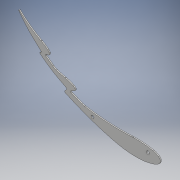
# Autodesk Inventor part: splitter
Saved by Autodesk Inventor 2018.3 (Build 223284000, 284)
## iProperties
Created: 2018-06-13
Part Number: splitter
Material: 一般
Document SubType Name: Modeling
Designer: ku_sk
Density: 1 g/cm^3
Appearance: 既定
Author: ku_sk
Autodesk Inventor part; units mm, degrees
ref_plane "YZ Plane" through (0, 0, 0) normal (1, 0, 0) x (0, 1, 0)
ref_plane "XZ Plane" through (0, 0, 0) normal (0, 1, 0) x (-1, 0, 0)
ref_plane "XY Plane" through (0, 0, 0) normal (0, 0, 1) x (1, 0, 0)
sketch "スケッチ1" plane through (0, 0, 0) normal (0, 1, 0) x (-1, 0, 0)
  circle A0 centre (32.803, 5.2135) radius 6 projected
  circle A1 centre (426.1472, 150.6128) radius 3 projected
  circle A2 centre (327.3904, 78.8305) radius 3 projected
  circle A3 centre (411.0696, 106.0665) radius 3 projected
  circle A4 centre (499.9259, 198.5785) radius 3 projected
  circle A5 centre (247.4696, 17.1833) radius 6 projected
  arc A6 (451.6654, 129.0808) -> (451.2836, 131.7777) centre (450.6431, 130.3115) ccw projected
  arc A7 (397.0782, 90.3195) -> (451.6654, 129.0808) centre (168.8146, 469.5991) ccw projected
  arc A8 (380.6202, 81.0666) -> (397.0782, 90.3195) centre (232.593, 363.6259) ccw projected
  line L0 (380.6202, 81.0666) -> (348.4629, 64.22) projected
  arc A9 (348.4629, 64.22) -> (347.5624, 59.6278) centre (349.8551, 61.5626) ccw projected
  line L1 (347.5624, 59.6278) -> (354.3249, 51.6146) projected
  arc A10 (352.9404, 45.4012) -> (354.3249, 51.6146) centre (351.268, 49.0348) ccw projected
  arc A11 (196.042, -12.8796) -> (352.9404, 45.4012) centre (-109.7603, 1050.7077) ccw projected
  arc A12 (150.312, -24.5744) -> (196.042, -12.8796) centre (-24.3171, 753.5344) ccw projected
  arc A13 (62.5903, -32.1265) -> (150.312, -24.5744) centre (78.6271, 294.8376) ccw projected
  arc A14 (7.8921, -21.3368) -> (62.5903, -32.1265) centre (71.9931, 159.5809) ccw projected
  arc A15 (-9.4003, -11.6891) -> (7.8921, -21.3368) centre (27.6212, 34.3463) ccw projected
  arc A16 (-8.119, 12.6128) -> (-9.4003, -11.6891) centre (0, 0) ccw projected
  arc A17 (11.7348, 20.8189) -> (-8.119, 12.6128) centre (24.3569, -37.8384) ccw projected
  arc A18 (90.7942, 27.108) -> (11.7348, 20.8189) centre (74.8452, -272.4677) ccw projected
  arc A19 (90.7942, 27.108) -> (95.7842, 26.8528) centre (154.5899, 1225.411) ccw projected
  arc A20 (95.7842, 26.8528) -> (277.8916, 37.5161) centre (137.4382, 875.8316) ccw projected
  arc A21 (277.8916, 37.5161) -> (287.7058, 40.2106) centre (269.6296, 86.8287) ccw projected
  line L2 (287.7058, 40.2106) -> (329.9476, 56.5899) projected
  arc A22 (329.9476, 56.5899) -> (330.1161, 63.979) centre (328.5015, 60.3193) ccw projected
  line L3 (330.1161, 63.979) -> (317.5781, 69.5105) projected
  arc A23 (315.5573, 79.0327) -> (317.5781, 69.5105) centre (320, 75) ccw projected
  arc A24 (322.3786, 84.2587) -> (315.5573, 79.0327) centre (333.3281, 62.902) ccw projected
  arc A25 (352.2737, 94.8734) -> (322.3786, 84.2587) centre (377.1259, -22.5249) ccw projected
  arc A26 (352.2737, 94.8734) -> (354.2282, 95.2914) centre (252.865, 564.4668) ccw projected
  arc A27 (354.2282, 95.2914) -> (387.5718, 104.2897) centre (282.4293, 427.624) ccw projected
  arc A28 (387.5718, 104.2897) -> (401.6356, 111.4877) centre (372.1097, 151.8389) ccw projected
  line L4 (401.6356, 111.4877) -> (428.0001, 130.7792) projected
  arc A29 (428.0001, 130.7792) -> (426.2504, 137.9601) centre (425.638, 134.0073) ccw projected
  line L5 (426.2504, 137.9601) -> (419.0814, 139.0707) projected
  arc A30 (414.665, 147.7454) -> (419.0814, 139.0707) centre (420, 145) ccw projected
  arc A31 (419.9012, 154.5588) -> (414.665, 147.7454) centre (436.0051, 136.7638) ccw projected
  arc A32 (446.0304, 172.5493) -> (419.9012, 154.5588) centre (500.4207, 65.5835) ccw projected
  arc A33 (446.0304, 172.5493) -> (447.8101, 173.4589) centre (228.4693, 600.4128) ccw projected
  arc A34 (447.8101, 173.4589) -> (530.7544, 233.381) centre (292.4437, 475.8846) ccw projected
  arc A35 (533.1819, 231.3155) -> (530.7544, 233.381) centre (531.8758, 232.2398) ccw projected
  arc A36 (490.4869, 179.7468) -> (533.1819, 231.3155) centre (171.8364, 487.0238) ccw projected
  arc A37 (476.9845, 166.5496) -> (490.4869, 179.7468) centre (260.8694, 401.1686) ccw projected
  line L6 (476.9845, 166.5496) -> (446.4931, 138.463) projected
  arc A38 (446.4931, 138.463) -> (447.3246, 133.5074) centre (448.5256, 136.2565) ccw projected
  line L7 (447.3246, 133.5074) -> (451.2836, 131.7777) projected
  point P0 (0, 0)
extrude "押し出し1" add sketch "スケッチ1" along normal mid plane 4 contours A1 | A2 | A3 | A4 | A7 A8 L0 A9 L1 A10 A11 A12 A13 A14 A15 A16 A17 A18 A19 A20 A21 L2 A22 L3 A23 A24 A25 A26 A27 A28 L4 A29 L5 A30 A31 A32 A33 A34 A35 A36 A37 L6 A38 L7 A6
